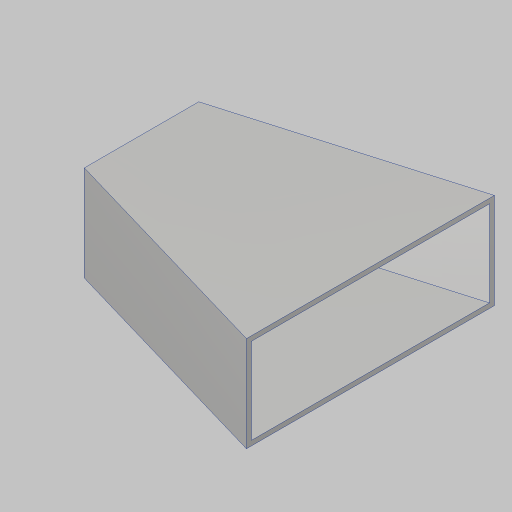
# Autodesk Inventor part: feeder block
Saved by Autodesk Inventor 2023.5 (Build 275446000, 446)
## iProperties
Created: 2025-01-16
Part Number: feeder block
Material: Aluminum 6061
Document SubType Name: Modeling
Designer: slick
Density: 2.7 g/cm^3
Appearance: Aluminum - Flat
Author: slick
Autodesk Inventor part; units mm, degrees
ref_plane "YZ Plane" through (0, 0, 0) normal (1, 0, 0) x (0, 1, 0)
ref_plane "XZ Plane" through (0, 0, 0) normal (0, 1, 0) x (-1, 0, 0)
ref_plane "XY Plane" through (0, 0, 0) normal (0, 0, 1) x (1, 0, 0)
sketch "Sketch1" plane through (0, 0, 0) normal (0, 1, 0) x (-1, 0, 0)
  line L0 (0, 165.1) -> (304.8, 76.2)
  line L1 (304.8, 76.2) -> (304.8, -76.2)
  line L2 (304.8, -76.2) -> (0, -165.1)
  line L3 (0, -165.1) -> (0, 165.1)
  point P0 (0, 0)
  point P1 (304.8, 0)
  point P2 (0, 0)
  dimension "d0" = 330.2
  dimension "d1" = 152.4
  dimension "d2" = 304.8
  constraints: 8 end point, 2 midpoint, 1 coincident, 1 horizontal alignment, 1 parallel, 1 vertical
  measures "d0" distance of L2.end L0.start
  measures "d1" distance of L0.end L1.end
  measures "d2" distance between parallel lines of L3 L1
extrude "Extrusion1" add sketch "Sketch1" along normal blind 127
shell "Shell1" thickness 6.35 removed faces 2 at (0, 42.3333, 55.0333) at (-304.8, 42.3333, -25.4)
body "Solid1"
